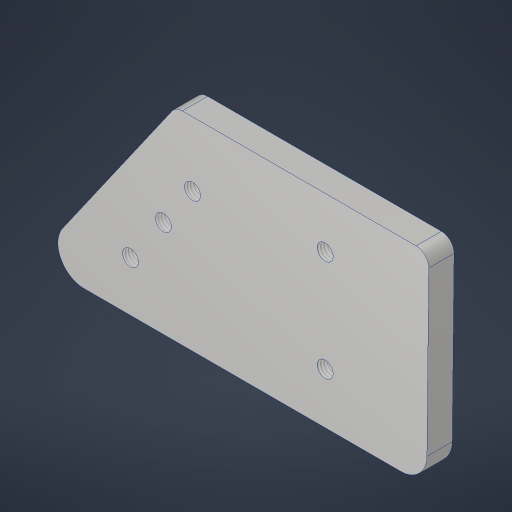
# Autodesk Inventor part: CL7-011
Saved by Autodesk Inventor 2023.4 (Build 274418000, 418)
## iProperties
Created: 2025-03-18
Part Number: CL7-011
Material: Aluminum 6061
Document SubType Name: Modeling
Designer: slick
Density: 2.7 g/cm^3
Appearance: Aluminum - Flat
Author: slick
Autodesk Inventor part; units mm, degrees
ref_plane "YZ Plane" through (0, 0, 0) normal (1, 0, 0) x (0, 1, 0)
ref_plane "XZ Plane" through (0, 0, 0) normal (0, 1, 0) x (-1, 0, 0)
ref_plane "XY Plane" through (0, 0, 0) normal (0, 0, 1) x (1, 0, 0)
sketch "Sketch1" plane through (0, 0, 0) normal (0, 0, 1) x (1, 0, 0)
  line L0 (0, 0) -> (50.8, 0) construction
  line L1 (50.8, 0) -> (50.8, 387.35) construction
  line L2 (50.8, 387.35) -> (0, 387.35) construction
  line L3 (0, 387.35) -> (0, 0) construction
  line L4 (20.8065, 339.141) -> (-226.8638, -14.5688) construction
  line L5 (-226.8638, -14.5688) -> (-247.6703, 0) construction
  line L6 (-247.6703, 0) -> (0, 353.7099) construction
  line L7 (0, 353.7099) -> (20.8065, 339.141) construction
  line L8 (-247.6703, 0) -> (-216.6626, 0) construction
  line L9 (0, 353.7099) -> (0, 309.4263) construction
  dimension "d0" = 50.8
  dimension "d1" = 387.35
  dimension "d2" = 25.4
  dimension "d3" = 431.8
  dimension "d5" = 55
  constraints: 20 end point, 4 parallel, 2 horizontal, 2 perpendicular, 2 point on line, 1 horizontal alignment, 1 vertical, 1 vertical alignment
  measures "d0" distance of L2.end L1.end
  measures "d1" distance of L1.end L0.end
  measures "d2" distance of L4.end L5.end
  measures "d3" distance of L5.end L6.end
  measures "d5" angle of L7 L3
sketch "Sketch2" plane through (0, 0, 0) normal (0, 0, 1) x (1, 0, 0)
  line L0 (0, 0) -> (50.8, 0) construction
  line L1 (50.8, 0) -> (50.8, 387.35) construction
  line L2 (50.8, 387.35) -> (0, 387.35) construction
  line L3 (0, 387.35) -> (0, 0) construction
  line L4 (20.8065, 339.141) -> (-226.8638, -14.5688) construction
  line L5 (-226.8638, -14.5688) -> (-247.6703, 0) construction
  line L6 (-247.6703, 0) -> (0, 353.7099) construction
  line L7 (0, 353.7099) -> (20.8065, 339.141) construction
  line L8 (-247.6703, 0) -> (-216.6626, 0) construction
  line L9 (0, 353.7099) -> (0, 309.4263) construction
  circle A0 centre (12.7, 431.8) radius 11.176
  circle A1 centre (12.7, 431.8) radius 23.8125 construction
  circle A2 centre (12.7, 431.8) radius 39.6875 construction
  line L10 (-47.586, 285.75) -> (0, 353.7099)
  line L11 (0, 387.35) -> (0, 353.7099)
  line L12 (0, 387.35) -> (-16.2292, 404.6302)
  line L13 (52.3851, 431.368) -> (50.8, 285.75)
  line L14 (50.8, 285.75) -> (-47.586, 285.75)
  arc A3 (52.3851, 431.368) -> (-16.2292, 404.6302) centre (12.7, 431.8) ccw
  line L15 (12.7, 374.65) -> (38.1, 374.65) construction
  line L16 (10.4032, 346.4254) -> (-237.2671, -7.2844) construction
  point P0 (25.4, 0)
  point P1 (-7.8078, 320.4174)
  point P2 (-15.0922, 310.0141)
  point P3 (-23.3303, 298.2489)
  point P4 (25.4, 374.65)
  point P5 (25.4, 374.65)
  point P6 (25.4, 387.35)
  dimension "d6" = 22.352
  dimension "d7" = 47.625
  dimension "d8" = 15.875
  dimension "d10" = 12.7
  dimension "d11" = 431.8
  dimension "d12" = 101.6
  dimension "d13" = 25.4
  dimension "d14" = 12.7
  dimension "d15" = 12.7
  dimension "d16" = 14.3627
  dimension "d56" = 31.75
  constraints: 14 end point, 5 midpoint, 5 point on line, 4 centre point, 4 point on circle, 3 coincident, 2 perpendicular, 2 tangent, 1 collinear, 1 horizontal, 1 vertical alignment
  measures "d6" diameter of A0
  measures "d7" diameter of A1
  measures "d8" radial gap between concentric circles of A1 A2
  measures "d10" distance from line of L3 A0.centre
  measures "d11" distance from line of L0 A0.centre
  measures "d12" distance between parallel lines of L2 L14
  measures "d13" distance of L15.start L15.end
  measures "d14" distance between parallel lines of L2 L15
  measures "d15" distance of point (-15.092, 310.014) point (-7.808, 320.417)
  measures "d16" distance of point (-15.092, 310.014) point (-23.33, 298.249)
  measures "d56" distance from line of point (-7.808, 320.417) L7
extrude "Extrusion1" add sketch "Sketch2" along normal blind 6.35
hole "Hole1" at (0, 0, 0) at (50.8, 0, 0) at (-226.8638, -14.5688, 0) at (-247.6703, 0, 0) at (-216.6626, 0, 0) at (-7.8078, 320.4174, 0) at (-15.0922, 310.0141, 0) at (-23.3303, 298.2489, 0) at (12.7, 374.65, 0) at (25.4, 374.65, 0) at (38.1, 374.65, 0) direction (0, 0, 1) diameter 3.9624 end through all thread size "10-32 UNF" class "2B" standard "ANSI Unified Screw Threads"
fillet "Fillet1" radius 6.604 3 edges at (0, 353.7099, 3.175) (-47.586, 285.75, 3.175) (50.8, 285.75, 3.175)
sketch "Sketch3" plane through (0, 0, 0) normal (0, 0, -1) x (-1, 0, 0)
  arc A0 (-50.8711, 292.2821) -> (-44.2675, 285.75) centre (-44.2675, 292.354) ccw construction
  line L0 (34.8998, 285.75) -> (-44.2675, 285.75) construction
  arc A1 (34.8998, 285.75) -> (40.3095, 296.1419) centre (34.8998, 292.354) ccw construction
  line L1 (1.1943, 352.0042) -> (40.3095, 296.1419) construction
  arc A2 (0, 355.7921) -> (1.1943, 352.0042) centre (6.604, 355.7921) ccw construction
  line L2 (0, 387.35) -> (0, 355.7921) construction
  line L3 (16.2292, 404.6302) -> (0, 387.35) construction
  arc A3 (16.2292, 404.6302) -> (-52.3851, 431.368) centre (-12.7, 431.8) ccw construction
  line L4 (-50.8711, 292.2821) -> (-52.3851, 431.368) construction
  circle A4 centre (-25.4, 374.65) radius 1.9812 construction
  circle A5 centre (23.3303, 298.2489) radius 1.9812 construction
  circle A6 centre (7.8078, 320.4174) radius 1.9812 construction
  circle A7 centre (15.0922, 310.0141) radius 1.9812 construction
  circle A8 centre (-12.7, 374.65) radius 1.9812 construction
  circle A9 centre (-38.1, 374.65) radius 1.9812 construction
  circle A10 centre (-12.7, 431.8) radius 11.176 construction
  circle A11 centre (-12.7, 431.8) radius 23.8125
  circle A12 centre (-12.7, 431.8) radius 11.176 construction
  circle A13 centre (-12.7, 431.8) radius 31.75 construction
  point P0 (0, 0)
  point P1 (-12.7, 463.55)
  point P2 (-44.45, 431.8)
  point P3 (-12.7, 400.05)
  point P4 (19.05, 431.8)
  dimension "d29" = 63.5
  dimension "d28" = 47.625
  dimension "d32" = 360
  constraints: 2 coincident, 2 vertical alignment, 1 centre point, 7 other
  measures "d28" diameter of A11
extrude "Extrusion2" cut sketch "Sketch3" against normal blind 3.175
hole "Hole2" at (12.7, 463.55, 0) at (44.45, 431.8, 0) at (12.7, 400.05, 0) at (-19.05, 431.8, 0) direction (0, 0, 1) diameter 3.9624 end through all thread size "10-32 UNF" class "2B" standard "ANSI Unified Screw Threads"
sketch "Sketch4" plane through (0, 0, 6.35) normal (0, 0, 1) x (1, 0, 0)
  line L0 (-1.1943, 352.0042) -> (-40.3095, 296.1419) projected
  line L1 (-12.0155, 336.55) -> (51.353, 336.55)
  line L2 (50.8711, 292.2821) -> (52.3851, 431.368) projected
  line L3 (-34.8998, 285.75) -> (44.2675, 285.75) projected
  arc A0 (-40.3095, 296.1419) -> (-34.8998, 285.75) centre (-34.8998, 292.354) ccw projected
  arc A1 (44.2675, 285.75) -> (50.8711, 292.2821) centre (44.2675, 292.354) ccw projected
  point P0 (0, 0)
  dimension "d43" = 50.8
  constraints: 2 end point, 2 point on line, 1 horizontal
  measures "d43" distance between parallel lines of L3 L1
extrude "Extrusion3" cut sketch "Sketch4" against normal through all keep common part
fillet "Fillet2" radius 3.175 2 edges at (-12.0155, 336.55, 3.175) (51.353, 336.55, 3.175)
sketch "Sketch5" plane through (0, 0, 6.35) normal (0, 0, 1) x (1, 0, 0)
  line L0 (50.8, 387.35) -> (0, 387.35) construction
  line L1 (25.4, 323.85) -> (25.4, 298.45) construction
  line L2 (-34.8998, 285.75) -> (44.2675, 285.75) construction
  point P0 (0, 0)
  point P1 (25.4, 387.35)
  dimension "d47" = 25.4
  dimension "d48" = 12.7
  constraints: 2 end point, 2 vertical alignment, 1 midpoint, 1 vertical
  measures "d47" distance of L1.start L1.end
  measures "d48" distance from line of L2 L1.end
hole "Hole3" at (25.4, 323.85, 6.35) at (25.4, 298.45, 6.35) direction (0, 0, -1) diameter 3.9624 end through all thread size "10-32 UNF" class "2B" standard "ANSI Unified Screw Threads"
body "Solid1"
